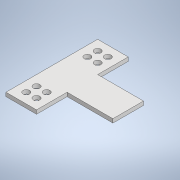
# Autodesk Inventor part: Lift.03.02.00.01
Saved by Autodesk Inventor 2021 (Build 250183000, 183)
## iProperties
Created: 2020-09-20
Part Number: Lift.03.02.00.01
Material: Типовые
Document SubType Name: ЛистМат
Designer: Kostya
Density: 1 g/cm^3
Sheet Metal Rule: По умолчанию_мм
Appearance: По умолчанию
Author: Kostya
Autodesk Inventor part; units mm, degrees
ref_plane "YZ Plane" through (0, 0, 0) normal (1, 0, 0) x (0, 1, 0)
ref_plane "XZ Plane" through (0, 0, 0) normal (0, 1, 0) x (-1, 0, 0)
ref_plane "XY Plane" through (0, 0, 0) normal (0, 0, 1) x (1, 0, 0)
sketch "Эскиз1" plane through (0, 0, 0) normal (0, 1, 0) x (-1, 0, 0)
  line L0 (118.3558, 0) -> (-118.3558, 0) construction
  line L1 (80, 0) -> (80, 120)
  line L2 (80, 120) -> (0, 120)
  line L3 (0, 120) -> (0, 40)
  line L4 (0, 40) -> (-120, 40)
  line L5 (-120, 40) -> (-120, 0)
  circle A0 centre (53.3333, 93.3333) radius 8.5
  circle A1 centre (53.3333, 66.6667) radius 8.5
  circle A2 centre (26.6667, 93.3333) radius 8.5
  circle A3 centre (26.6667, 66.6667) radius 8.5
  line L6 (0, 40) -> (80, 40) construction
  line L7 (80, 0) -> (80, -120)
  line L8 (80, -120) -> (0, -120)
  line L9 (0, -120) -> (0, -40)
  line L10 (0, -40) -> (-120, -40)
  line L11 (-120, -40) -> (-120, 0)
  circle A4 centre (53.3333, -93.3333) radius 8.5
  circle A5 centre (53.3333, -66.6667) radius 8.5
  circle A6 centre (26.6667, -93.3333) radius 8.5
  circle A7 centre (26.6667, -66.6667) radius 8.5
  line L12 (0, -40) -> (80, -40) construction
  point P0 (0, 0)
  point P1 (0, 0)
  dimension "d0" = 200
  dimension "d1" = 80
  dimension "d2" = 80
  dimension "d3" = 120
  dimension "d5" = 17
  dimension "d7" = 26.6667
  dimension "d8" = 26.6667
  dimension "d9" = 26.6667
  dimension "d10" = 26.6667
  measures "d0" distance between parallel lines of L5 L1
  measures "d1" distance of L1.end L2.end
  measures "d2" distance of L2.end L3.end
  measures "d3" distance between parallel lines of L0 L2
  measures "d5" diameter of A2
  measures "d7" distance from line of A0.centre L1
  measures "d8" distance of A2.centre A0.centre
  measures "d9" distance from line of L2 A0.centre
  measures "d10" distance of A1.centre A0.centre
extrude "Пластина1" add sketch "Эскиз1" along normal blind 10
equation "\"d8\" = d7"
equation "\"d9\" = d7"
equation "\"d10\" = d9"
equation "\"d11\" = Толщина"
equation "\"Глубина_просечки\" = 0.5 * Толщина"
equation "\"Толщина\" = 10"
